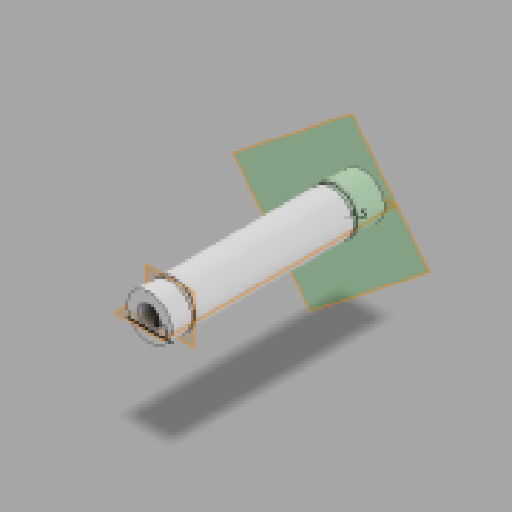
# Autodesk Inventor part: Вал 2 оси
Saved by Autodesk Inventor 2025 (Build 290162000, 162)
## iProperties
Created: 2025-04-09
Part Number: Вал 2 оси
Material: Типовые
Document SubType Name: Modeling
Designer: Artem Sannikov
Density: 1 g/cm^3
Appearance: По умолчанию
Author: Artem Sannikov
Autodesk Inventor part; units mm, degrees
ref_plane "YZ Plane" through (0, 0, 0) normal (1, 0, 0) x (0, 1, 0)
ref_plane "XY Plane" through (0, 0, 0) normal (0, 0, 1) x (1, 0, 0)
sketch "Эскиз1" plane through (0, 0, 0) normal (0, 0, 1) x (1, 0, 0)
  circle A0 centre (0, 3) radius 3 projected
  circle A1 centre (0, 3) radius 6
  point P0 (0, 0)
  dimension "d0" = 12
  constraints: 1 centre point, 1 coincident, 1 vertical alignment
  measures "d0" diameter of A1
extrude "Выдавливание1" add sketch "Эскиз1" along normal blind 58
sketch "Эскиз2" plane through (0, 0, 0) normal (0, 1, 0) x (-1, 0, 0)
  line L0 (6, 58) -> (-6, 58) projected
  line L1 (0, 58) -> (0, 55) construction
  line L2 (0, 0) -> (0, 4.5)
  dimension "d4" = 3
  dimension "d5" = 4.5
  constraints: 4 end point, 2 coincident, 2 vertical, 1 midpoint
  measures "d4" distance of L1.start L1.end
  measures "d5" distance of L2.start L2.end
ref_plane "РабПлоскость1" through (0, 2.25, 0) normal (0, 1, 0) x (-1, 0, 0)
sketch "Эскиз3" plane through (0, 2.25, 0) normal (0, 1, 0) x (-1, 0, 0)
  point P0 (0, 0)
  point P1 (0, 55)
  point P2 (0, 4.5)
hole "Отверстие1" at (0, 2.25, 55) at (0, 2.25, 4.5) direction (0, -1, 0) diameter 2.459 depth 8.8 tip angle 118 thread size "M3x0.5" class "6H" standard "ISO Metric profile"
ref_plane "РабПлоскость2" through (0, 3, 52.5) normal (0, 0, 1) x (1, 0, 0)
sketch "Эскиз4" plane through (0, 3, 52.5) normal (0, 0, 1) x (1, 0, 0)
  circle A0 centre (0, 0) radius 5.65
  circle A1 centre (0, 0) radius 6.8955
  point P0 (0, -3)
  dimension "d15" = 11.3
  constraints: 2 centre point, 1 coincident
  measures "d15" diameter of A0
extrude "Выдавливание2" cut sketch "Эскиз4" against normal blind 1.2
ref_plane "РабПлоскость3" through (0, 3, 8.5) normal (0, 0, -1) x (0.7866, 0.6175, 0)
sketch "Эскиз5" plane through (0, 3, 8.5) normal (0, 0, -1) x (0.7866, 0.6175, 0)
  circle A0 centre (0, 0) radius 5.65
  circle A1 centre (0, 0) radius 6.969
  point P0 (-1.8524, 2.3598)
  dimension "d18" = 11.3
  constraints: 2 centre point, 1 coincident
  measures "d18" diameter of A0
extrude "Выдавливание3" cut sketch "Эскиз5" along normal blind 1.2
ref_plane "РабПлоскость4" through (6.468, -1.8388, 51.5) normal (-0.6175, 0.7866, 0) x (0.7866, 0.6175, 0)
sketch "Эскиз6" plane through (6.468, -1.8388, 51.5) normal (-0.6175, 0.7866, 0) x (0.7866, 0.6175, 0)
  line L0 (-8.1, -6.5) -> (3.9, -6.5) projected
  line L1 (-2.1, -6.5) -> (-2.1, 51.5) construction
  line L2 (-8.1, 51.5) -> (3.9, 51.5) projected
  line L3 (-2.1, 3.542) -> (-2.1, 39.542) construction
  line L4 (-0.1, 3.542) -> (-0.1, 39.542)
  line L5 (-4.1, 39.542) -> (-4.1, 3.542)
  arc A0 (-4.1, 3.542) -> (-0.1, 3.542) centre (-2.1, 3.542) ccw
  arc A1 (-0.1, 39.542) -> (-4.1, 39.542) centre (-2.1, 39.542) ccw
  point P0 (-3.9524, 51.5)
  point P1 (-2.1, 21.542)
  dimension "d21" = 36
  dimension "d22" = 4
  constraints: 10 end point, 4 point on circle, 4 tangent, 3 midpoint, 2 centre point, 2 point on line, 1 parallel
  measures "d21" distance of L3.start L3.end
  measures "d22" diameter of A1
extrude "Выдавливание4" cut sketch "Эскиз6" along normal blind 4.3
